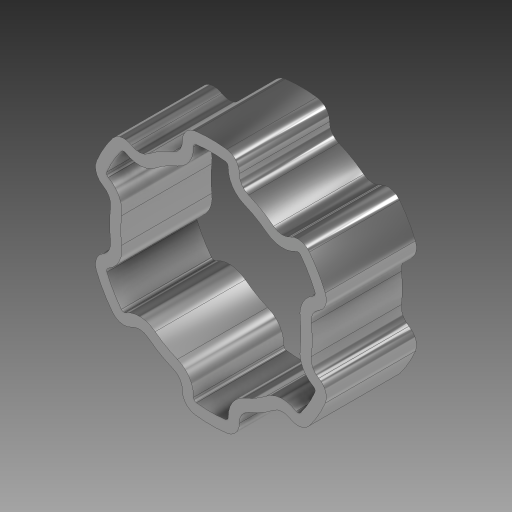
# Autodesk Inventor part: MAXTube
Saved by Autodesk Inventor 2024 (Build 280153000, 153)
## iProperties
Created: 2022-12-09
Part Number: MAXTube
Material: Aluminum 6061
Document SubType Name: Modeling
Designer: Max Boord
Density: 2.7 g/cm^3
Appearance: Chrome - Polished Black
Mass: 6.07807 g
Surface Area: 32.131 cm^2
Volume: 2.25114 cm^3
Mass: 218.811 g
Surface Area: 1032.64 cm^2
Volume: 81.0409 cm^3
Author: Max Boord
Mass: 226.408 g
Surface Area: 1068.37 cm^2
Volume: 83.8549 cm^3
Mass: 220.33 g
Surface Area: 1039.78 cm^2
Volume: 81.6037 cm^3
Mass: 224.889 g
Surface Area: 1061.22 cm^2
Volume: 83.2921 cm^3
Autodesk Inventor part; units mm, degrees
ref_plane "YZ Plane" through (0, 0, 0) normal (1, 0, 0) x (0, 1, 0)
ref_plane "XZ Plane" through (0, 0, 0) normal (0, 1, 0) x (-1, 0, 0)
ref_plane "XY Plane" through (0, 0, 0) normal (0, 0, 1) x (1, 0, 0)
sketch "MaxSpline" plane through (0, 0, 0) normal (0, 0, 1) x (1, 0, 0)
  line L0 (0, 0) -> (0, 22.7025) construction
  line L1 (-1.9737, 15.2856) -> (0, 0) construction
  line L2 (1.9737, 15.2856) -> (0, 0) construction
  line L3 (-10.0992, 12.8421) -> (0, 0) construction
  line L4 (-6.072, 15.1672) -> (0, 0) construction
  arc A0 (2.2346, 17.3063) -> (-2.2346, 17.3063) centre (0, 0) ccw
  arc A1 (16.105, 6.718) -> (13.8704, 10.5884) centre (0, 0) ccw
  arc A2 (13.8704, -10.5884) -> (16.105, -6.718) centre (0, 0) ccw
  arc A3 (-2.2346, -17.3063) -> (2.2346, -17.3063) centre (0, 0) ccw
  arc A4 (-13.8704, 10.5884) -> (-16.105, 6.718) centre (0, 0) ccw
  arc A5 (-16.105, -6.718) -> (-13.8704, -10.5884) centre (0, 0) ccw
  arc A6 (14.1297, -2.0316) -> (14.1297, 2.0316) centre (0, 0) ccw
  arc A7 (5.3054, -13.2525) -> (8.8243, -11.2209) centre (0, 0) ccw
  arc A8 (-8.8243, -11.2209) -> (-5.3054, -13.2525) centre (0, 0) ccw
  arc A9 (-14.1297, 2.0316) -> (-14.1297, -2.0316) centre (0, 0) ccw
  arc A10 (-5.3054, 13.2525) -> (-8.8243, 11.2209) centre (0, 0) ccw
  arc A11 (8.8243, 11.2209) -> (5.3054, 13.2525) centre (0, 0) ccw
  arc A12 (-4.7209, 11.79) -> (-2.436, 15.2723) centre (-6.072, 15.1672) ccw
  arc A13 (-2.0329, 15.7443) -> (-2.436, 15.2723) centre (-1.9737, 15.2856) ccw
  arc A14 (2.0329, 15.7443) -> (-2.0329, 15.7443) centre (0, 0) ccw
  arc A15 (2.436, 15.2723) -> (2.0329, 15.7443) centre (1.9737, 15.2856) ccw
  arc A16 (2.436, 15.2723) -> (4.7201, 11.7903) centre (6.072, 15.1672) ccw
  arc A17 (7.8507, 9.9828) -> (4.7201, 11.7903) centre (0, 0) ccw
  arc A18 (7.8507, 9.9828) -> (12.0082, 9.7457) centre (10.0992, 12.8421) ccw
  arc A19 (12.6185, 9.6327) -> (12.0082, 9.7457) centre (12.2509, 9.3521) ccw
  arc A20 (14.6514, 6.1116) -> (12.6185, 9.6327) centre (0, 0) ccw
  arc A21 (14.4442, 5.5265) -> (14.6514, 6.1116) centre (14.2246, 5.9336) ccw
  arc A22 (14.4442, 5.5265) -> (12.5707, 1.8075) centre (16.1712, 2.3251) ccw
  arc A23 (12.5707, -1.8075) -> (12.5707, 1.8075) centre (0, 0) ccw
  arc A24 (12.5707, -1.8075) -> (14.4442, -5.5265) centre (16.1712, -2.3251) ccw
  arc A25 (14.6514, -6.1116) -> (14.4442, -5.5265) centre (14.2246, -5.9336) ccw
  arc A26 (12.6185, -9.6327) -> (14.6514, -6.1116) centre (0, 0) ccw
  arc A27 (12.0082, -9.7457) -> (12.6185, -9.6327) centre (12.2509, -9.3521) ccw
  arc A28 (12.0082, -9.7457) -> (7.8507, -9.9828) centre (10.0992, -12.8421) ccw
  arc A29 (4.7201, -11.7903) -> (7.8507, -9.9828) centre (0, 0) ccw
  arc A30 (4.7201, -11.7903) -> (2.436, -15.2723) centre (6.072, -15.1672) ccw
  arc A31 (2.0329, -15.7443) -> (2.436, -15.2723) centre (1.9737, -15.2856) ccw
  arc A32 (-2.0329, -15.7443) -> (2.0329, -15.7443) centre (0, 0) ccw
  arc A33 (-2.436, -15.2723) -> (-2.0329, -15.7443) centre (-1.9737, -15.2856) ccw
  arc A34 (-2.436, -15.2723) -> (-4.7201, -11.7903) centre (-6.072, -15.1672) ccw
  arc A35 (-7.8507, -9.9828) -> (-4.7201, -11.7903) centre (0, 0) ccw
  arc A36 (-7.8507, -9.9828) -> (-12.0082, -9.7457) centre (-10.0992, -12.8421) ccw
  arc A37 (-12.6185, -9.6327) -> (-12.0082, -9.7457) centre (-12.2509, -9.3521) ccw
  arc A38 (-14.6514, -6.1116) -> (-12.6185, -9.6327) centre (0, 0) ccw
  arc A39 (-14.4442, -5.5265) -> (-14.6514, -6.1116) centre (-14.2246, -5.9336) ccw
  arc A40 (-14.4442, -5.5265) -> (-12.5707, -1.8075) centre (-16.1712, -2.3251) ccw
  arc A41 (-12.5707, 1.8075) -> (-12.5707, -1.8075) centre (0, 0) ccw
  arc A42 (-12.5707, 1.8075) -> (-14.4442, 5.5265) centre (-16.1712, 2.3251) ccw
  arc A43 (-14.6514, 6.1116) -> (-14.4442, 5.5265) centre (-14.2246, 5.9336) ccw
  arc A44 (-12.6185, 9.6327) -> (-14.6514, 6.1116) centre (0, 0) ccw
  arc A45 (-12.0082, 9.7457) -> (-12.6185, 9.6327) centre (-12.2509, 9.3521) ccw
  arc A46 (-12.0082, 9.7457) -> (-7.8507, 9.9828) centre (-10.0992, 12.8421) ccw
  arc A47 (-4.7172, 11.7914) -> (-7.8507, 9.9828) centre (0, 0) ccw
  dimension "d10" = 14.715
  dimension "d11" = 16.364
  dimension "d13" = 34.9
  dimension "d14" = 28.55
  dimension "d15" = 25.4
  measures "d10" angle of L2 L1
  measures "d11" angle of L3 L4
  measures "d13" diameter of A0
  measures "d14" diameter of A11
  measures "d15" diameter of A17
sketch "Sketch1" plane through (0, 0, 0) normal (0, 0, 1) x (1, 0, 0)
  arc A0 (-2.2346, 17.3063) -> (-4.0103, 15.2268) centre (-1.9737, 15.2856) ccw
  arc A1 (-5.3054, 13.2525) -> (-4.0103, 15.2268) centre (-6.072, 15.1672) ccw
  arc A2 (4.0103, 15.2268) -> (2.2346, 17.3063) centre (1.9737, 15.2856) ccw
  arc A3 (4.0103, 15.2268) -> (5.3054, 13.2525) centre (6.072, 15.1672) ccw
  arc A4 (-16.105, 6.718) -> (-15.1919, 4.1403) centre (-14.2246, 5.9336) ccw
  arc A5 (-14.1297, 2.0316) -> (-15.1919, 4.1403) centre (-16.1712, 2.3251) ccw
  arc A6 (-11.1816, 11.0864) -> (-13.8704, 10.5884) centre (-12.2509, 9.3521) ccw
  arc A7 (-11.1816, 11.0864) -> (-8.8243, 11.2209) centre (-10.0992, 12.8421) ccw
  arc A8 (-13.8704, -10.5884) -> (-11.1816, -11.0864) centre (-12.2509, -9.3521) ccw
  arc A9 (-8.8243, -11.2209) -> (-11.1816, -11.0864) centre (-10.0992, -12.8421) ccw
  arc A10 (-15.1919, -4.1403) -> (-16.105, -6.718) centre (-14.2246, -5.9336) ccw
  arc A11 (-15.1919, -4.1403) -> (-14.1297, -2.0316) centre (-16.1712, -2.3251) ccw
  arc A12 (2.2346, -17.3063) -> (4.0103, -15.2268) centre (1.9737, -15.2856) ccw
  arc A13 (5.3054, -13.2525) -> (4.0103, -15.2268) centre (6.072, -15.1672) ccw
  arc A14 (-4.0103, -15.2268) -> (-2.2346, -17.3063) centre (-1.9737, -15.2856) ccw
  arc A15 (-4.0103, -15.2268) -> (-5.3054, -13.2525) centre (-6.072, -15.1672) ccw
  arc A16 (16.105, -6.718) -> (15.1919, -4.1403) centre (14.2246, -5.9336) ccw
  arc A17 (14.1297, -2.0316) -> (15.1919, -4.1403) centre (16.1712, -2.3251) ccw
  arc A18 (11.1816, -11.0864) -> (13.8704, -10.5884) centre (12.2509, -9.3521) ccw
  arc A19 (11.1816, -11.0864) -> (8.8243, -11.2209) centre (10.0992, -12.8421) ccw
  arc A20 (13.8704, 10.5884) -> (11.1816, 11.0864) centre (12.2509, 9.3521) ccw
  arc A21 (8.8243, 11.2209) -> (11.1816, 11.0864) centre (10.0992, 12.8421) ccw
  arc A22 (15.1919, 4.1403) -> (16.105, 6.718) centre (14.2246, 5.9336) ccw
  arc A23 (15.1919, 4.1403) -> (14.1297, 2.0316) centre (16.1712, 2.3251) ccw
  line L0 (0, 0) -> (0, 22.7025) construction
  line L1 (-1.9737, 15.2856) -> (0, 0) construction
  line L2 (1.9737, 15.2856) -> (0, 0) construction
  line L3 (-10.0992, 12.8421) -> (0, 0) construction
  line L4 (-6.072, 15.1672) -> (0, 0) construction
  arc A24 (2.2346, 17.3063) -> (-2.2346, 17.3063) centre (0, 0) ccw
  arc A25 (16.105, 6.718) -> (13.8704, 10.5884) centre (0, 0) ccw
  arc A26 (13.8704, -10.5884) -> (16.105, -6.718) centre (0, 0) ccw
  arc A27 (-2.2346, -17.3063) -> (2.2346, -17.3063) centre (0, 0) ccw
  arc A28 (-13.8704, 10.5884) -> (-16.105, 6.718) centre (0, 0) ccw
  arc A29 (-16.105, -6.718) -> (-13.8704, -10.5884) centre (0, 0) ccw
  arc A30 (14.1297, -2.0316) -> (14.1297, 2.0316) centre (0, 0) ccw
  arc A31 (5.3054, -13.2525) -> (8.8243, -11.2209) centre (0, 0) ccw
  arc A32 (-8.8243, -11.2209) -> (-5.3054, -13.2525) centre (0, 0) ccw
  arc A33 (-14.1297, 2.0316) -> (-14.1297, -2.0316) centre (0, 0) ccw
  arc A34 (-5.3054, 13.2525) -> (-8.8243, 11.2209) centre (0, 0) ccw
  arc A35 (8.8243, 11.2209) -> (5.3054, 13.2525) centre (0, 0) ccw
  arc A36 (-4.7209, 11.79) -> (-2.436, 15.2723) centre (-6.072, 15.1672) ccw
  arc A37 (-2.0329, 15.7443) -> (-2.436, 15.2723) centre (-1.9737, 15.2856) ccw
  arc A38 (2.0329, 15.7443) -> (-2.0329, 15.7443) centre (0, 0) ccw
  arc A39 (2.436, 15.2723) -> (2.0329, 15.7443) centre (1.9737, 15.2856) ccw
  arc A40 (2.436, 15.2723) -> (4.7201, 11.7903) centre (6.072, 15.1672) ccw
  arc A41 (7.8507, 9.9828) -> (4.7201, 11.7903) centre (0, 0) ccw
  arc A42 (7.8507, 9.9828) -> (12.0082, 9.7457) centre (10.0992, 12.8421) ccw
  arc A43 (12.6185, 9.6327) -> (12.0082, 9.7457) centre (12.2509, 9.3521) ccw
  arc A44 (14.6514, 6.1116) -> (12.6185, 9.6327) centre (0, 0) ccw
  arc A45 (14.4442, 5.5265) -> (14.6514, 6.1116) centre (14.2246, 5.9336) ccw
  arc A46 (14.4442, 5.5265) -> (12.5707, 1.8075) centre (16.1712, 2.3251) ccw
  arc A47 (12.5707, -1.8075) -> (12.5707, 1.8075) centre (0, 0) ccw
  arc A48 (12.5707, -1.8075) -> (14.4442, -5.5265) centre (16.1712, -2.3251) ccw
  arc A49 (14.6514, -6.1116) -> (14.4442, -5.5265) centre (14.2246, -5.9336) ccw
  arc A50 (12.6185, -9.6327) -> (14.6514, -6.1116) centre (0, 0) ccw
  arc A51 (12.0082, -9.7457) -> (12.6185, -9.6327) centre (12.2509, -9.3521) ccw
  arc A52 (12.0082, -9.7457) -> (7.8507, -9.9828) centre (10.0992, -12.8421) ccw
  arc A53 (4.7201, -11.7903) -> (7.8507, -9.9828) centre (0, 0) ccw
  arc A54 (4.7201, -11.7903) -> (2.436, -15.2723) centre (6.072, -15.1672) ccw
  arc A55 (2.0329, -15.7443) -> (2.436, -15.2723) centre (1.9737, -15.2856) ccw
  arc A56 (-2.0329, -15.7443) -> (2.0329, -15.7443) centre (0, 0) ccw
  arc A57 (-2.436, -15.2723) -> (-2.0329, -15.7443) centre (-1.9737, -15.2856) ccw
  arc A58 (-2.436, -15.2723) -> (-4.7201, -11.7903) centre (-6.072, -15.1672) ccw
  arc A59 (-7.8507, -9.9828) -> (-4.7201, -11.7903) centre (0, 0) ccw
  arc A60 (-7.8507, -9.9828) -> (-12.0082, -9.7457) centre (-10.0992, -12.8421) ccw
  arc A61 (-12.6185, -9.6327) -> (-12.0082, -9.7457) centre (-12.2509, -9.3521) ccw
  arc A62 (-14.6514, -6.1116) -> (-12.6185, -9.6327) centre (0, 0) ccw
  arc A63 (-14.4442, -5.5265) -> (-14.6514, -6.1116) centre (-14.2246, -5.9336) ccw
  arc A64 (-14.4442, -5.5265) -> (-12.5707, -1.8075) centre (-16.1712, -2.3251) ccw
  arc A65 (-12.5707, 1.8075) -> (-12.5707, -1.8075) centre (0, 0) ccw
  arc A66 (-12.5707, 1.8075) -> (-14.4442, 5.5265) centre (-16.1712, 2.3251) ccw
  arc A67 (-14.6514, 6.1116) -> (-14.4442, 5.5265) centre (-14.2246, 5.9336) ccw
  arc A68 (-12.6185, 9.6327) -> (-14.6514, 6.1116) centre (0, 0) ccw
  arc A69 (-12.0082, 9.7457) -> (-12.6185, 9.6327) centre (-12.2509, 9.3521) ccw
  arc A70 (-12.0082, 9.7457) -> (-7.8507, 9.9828) centre (-10.0992, 12.8421) ccw
  arc A71 (-4.7172, 11.7914) -> (-7.8507, 9.9828) centre (0, 0) ccw
  point P0 (-4.7201, 11.7903)
  point P1 (-4.7209, 11.79)
  point P2 (2.2346, 17.3063)
  point P3 (-2.2346, 17.3063)
  point P4 (-5.3054, 13.2525)
  point P5 (-8.8243, 11.2209)
  point P6 (-14.1297, 2.0316)
  point P7 (-14.1297, -2.0316)
  point P8 (-13.8704, -10.5884)
  point P9 (-8.8243, -11.2209)
  point P10 (-5.3054, -13.2525)
  point P11 (-2.2346, -17.3063)
  point P12 (5.3054, -13.2525)
  point P13 (8.8243, -11.2209)
  point P14 (13.8704, -10.5884)
  point P15 (14.1297, -2.0316)
  point P16 (14.1297, 2.0316)
  point P17 (16.105, 6.718)
  point P18 (8.8243, 11.2209)
  point P19 (5.3054, 13.2525)
  dimension "d7" = 360
  dimension "d9" = 2.0375
  dimension "d12" = 2.0625
  constraints: 48 point on circle, 24 centre point, 1 horizontal alignment, 1 tangent, 96 other
  measures "d9" radius of A0
  measures "d12" radius of A1
extrude "Length" add sketch "Sketch1" along normal mid plane 12.7
body "Solid1"
